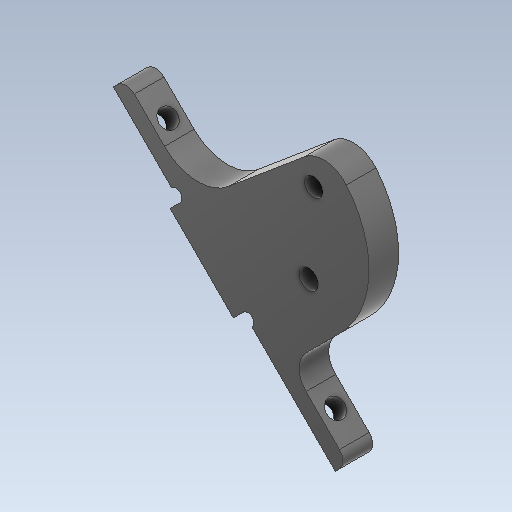
# Autodesk Inventor part: Camera_side_frame
Saved by Autodesk Inventor 2020.4 (Build 244396000, 396)
## iProperties
Created: 2021-09-12
Part Number: Camera_side_frame
Material: アセタール樹脂、黒
Document SubType Name: Modeling
Designer: t-nagamine
Density: 1.425 g/cm^3
Appearance: 滑らか - 黒
Description: POM T5
Mass: 5.16291 g
Surface Area: 23.9114 cm^2
Volume: 3.62309 cm^3
Author: Takuya Nagamine
Autodesk Inventor part; units mm, degrees
ref_plane "YZ Plane" through (0, 0, 0) normal (1, 0, 0) x (0, 1, 0)
ref_plane "XZ Plane" through (0, 0, 0) normal (0, 1, 0) x (-1, 0, 0)
ref_plane "XY Plane" through (0, 0, 0) normal (0, 0, 1) x (1, 0, 0)
derived "Head_side_frame.ipt"
sketch "スケッチ1" plane through (0, 0, 0) normal (0, 0, 1) x (1, 0, 0)
  line L0 (0, 0) -> (27, 0) construction
  line L1 (27, 0) -> (27, 5) construction
  line L2 (27, 5) -> (0, 5) construction
  line L3 (0, 5) -> (0, 0) construction
  line L4 (0, 2.5) -> (27, 2.5) construction
  line L5 (13.5, 5) -> (13.5, 0) construction
  circle A0 centre (3.7, 2.5) radius 1.55
  line L6 (7.5, 5) -> (7.5, 0) construction
  line L7 (19.5, 5) -> (19.5, 0) construction
  circle A1 centre (23.3, 2.5) radius 1.55
  line L8 (7.49, 5.01) -> (9.59, 5.01) construction
  line L9 (19.51, 5.01) -> (19.51, 2.49)
  line L10 (19.51, 2.49) -> (7.49, 2.49)
  line L11 (7.49, 2.49) -> (7.49, 5.01)
  line L12 (7.49, 5.01) -> (19.51, 2.49) construction
  line L13 (19.51, 5.01) -> (7.49, 2.49) construction
  arc A2 (9.59, 5.01) -> (7.49, 5.01) centre (8.54, 5.01) ccw
  arc A3 (19.51, 5.01) -> (17.41, 5.01) centre (18.46, 5.01) ccw
  line L14 (9.59, 5.01) -> (17.41, 5.01)
  line L15 (9.59, 2.49) -> (7.49, 2.49)
  line L16 (17.41, 5.01) -> (19.51, 5.01) construction
  line L17 (27, 7) -> (0, 7) construction
  line L18 (0, 0) -> (0, 7)
  line L19 (12.1912, 40) -> (12.1912, 35) construction
  circle A4 centre (14.8912, 37.5) radius 1.55
  line L20 (37.1912, 35) -> (37.1912, 40) construction
  line L21 (30.6912, 40) -> (30.6912, 35) construction
  circle A5 centre (34.4912, 37.5) radius 1.55
  line L22 (30.7012, 40.01) -> (30.7012, 34.99)
  line L23 (18.6912, 40) -> (18.6912, 35) construction
  line L24 (12.1912, 35) -> (37.1912, 35) construction
  line L25 (37.1912, 40) -> (12.1912, 40) construction
  line L26 (12.1912, 37.5) -> (37.1912, 37.5) construction
  line L27 (24.6912, 40) -> (24.6912, 35) construction
  line L28 (20.7812, 40.01) -> (28.6012, 40.01)
  line L29 (28.6012, 34.99) -> (20.7812, 34.99)
  line L30 (18.6812, 40.01) -> (30.7012, 34.99) construction
  line L31 (30.7012, 40.01) -> (18.6812, 34.99) construction
  arc A6 (30.7012, 40.01) -> (28.6012, 40.01) centre (29.6512, 40.01) ccw
  line L32 (28.6012, 40.01) -> (30.7012, 40.01) construction
  arc A7 (28.6012, 34.99) -> (30.7012, 34.99) centre (29.6512, 34.99) ccw
  line L33 (30.7012, 34.99) -> (28.6012, 34.99) construction
  line L34 (18.6812, 40.01) -> (20.7812, 40.01) construction
  line L35 (20.7812, 34.99) -> (18.6812, 34.99) construction
  arc A8 (20.7812, 40.01) -> (18.6812, 40.01) centre (19.7312, 40.01) ccw
  arc A9 (18.6812, 34.99) -> (20.7812, 34.99) centre (19.7312, 34.99) ccw
  line L36 (18.6812, 34.99) -> (18.6812, 40.01)
  line L37 (18.6912, 73) -> (18.6912, 68) construction
  line L38 (18.6812, 67.99) -> (18.6812, 73.01)
  line L39 (20.7812, 67.99) -> (18.6812, 67.99) construction
  arc A10 (18.6812, 67.99) -> (20.7812, 67.99) centre (19.7312, 67.99) ccw
  arc A11 (20.7812, 73.01) -> (18.6812, 73.01) centre (19.7312, 73.01) ccw
  line L40 (24.6912, 73) -> (24.6912, 68) construction
  line L41 (12.1912, 70.5) -> (37.1912, 70.5) construction
  line L42 (37.1912, 73) -> (12.1912, 73) construction
  line L43 (12.1912, 68) -> (37.1912, 68) construction
  line L44 (30.7012, 73.01) -> (18.6812, 67.99) construction
  line L45 (18.6812, 73.01) -> (30.7012, 67.99) construction
  line L46 (28.6012, 67.99) -> (20.7812, 67.99)
  line L47 (20.7812, 73.01) -> (28.6012, 73.01)
  line L48 (37.1912, 68) -> (37.1912, 73) construction
  line L49 (18.6812, 73.01) -> (20.7812, 73.01) construction
  line L50 (30.6912, 73) -> (30.6912, 68) construction
  arc A12 (30.7012, 73.01) -> (28.6012, 73.01) centre (29.6512, 73.01) ccw
  line L51 (28.6012, 73.01) -> (30.7012, 73.01) construction
  line L52 (30.7012, 73.01) -> (30.7012, 67.99)
  line L53 (30.7012, 67.99) -> (28.6012, 67.99) construction
  circle A13 centre (34.4912, 70.5) radius 1.55
  arc A14 (28.6012, 67.99) -> (30.7012, 67.99) centre (29.6512, 67.99) ccw
  circle A15 centre (14.8912, 70.5) radius 1.55
  line L54 (12.1912, 73) -> (12.1912, 68) construction
  line L55 (27, 0) -> (27, 6.6473)
  line L56 (37.1912, 35) -> (27.1206, 7.3314)
  line L57 (11.8992, 39.6929) -> (0, 7)
  line L58 (37.1912, 35) -> (37.1912, 73)
  line L59 (6.8054, 101.4338) -> (6.7491, 101.3865)
  arc A16 (4.7394, 86.3065) -> (5.3203, 95.7003) centre (-4.8938, 91.617) ccw
  circle A17 centre (-4.8938, 91.617) radius 14.6063 construction
  line L60 (1.0459, 61.9185) -> (-21.5815, 84.5459) construction
  line L61 (-21.5815, 84.5459) -> (-18.0459, 88.0815) construction
  line L62 (-18.0459, 88.0815) -> (4.5815, 65.4541) construction
  line L63 (4.5815, 65.4541) -> (1.0459, 61.9185) construction
  line L64 (1.0459, 61.9185) -> (-18.0459, 88.0815) construction
  line L65 (-21.5815, 84.5459) -> (4.5815, 65.4541) construction
  line L66 (13.8495, 100.8175) -> (37.1912, 73)
  arc A18 (11.8992, 39.6929) -> (5.2055, 80.7796) centre (-28.1256, 54.2607) ccw
  arc A19 (8.344, 97.7899) -> (6.2953, 101.0057) centre (-4.8938, 91.617) ccw construction
  arc A20 (5.0756, 80.942) -> (7.4988, 83.886) centre (-4.8938, 91.617) ccw construction
  circle A21 centre (8.344, 97.7899) radius 1.55
  circle A22 centre (7.4988, 83.886) radius 1.65
  arc A23 (13.8495, 100.8175) -> (6.8054, 101.4338) centre (10.0193, 97.6035) ccw
  arc A24 (6.7491, 101.3865) -> (5.3203, 95.7003) centre (9.9631, 97.5563) ccw
  arc A25 (4.7394, 86.3065) -> (5.2055, 80.7796) centre (9.1182, 83.8926) ccw
  arc A26 (27.1206, 7.3314) -> (27, 6.6473) centre (29, 6.6473) ccw
  arc A27 (7.49, 3.9749) -> (8.9749, 2.49) centre (8.2325, 3.2325) ccw
  arc A28 (18.0251, 2.49) -> (19.51, 3.9749) centre (18.7675, 3.2325) ccw
  line L67 (0, 0) -> (7.5, -0.5)
  line L68 (7.5, -0.5) -> (19.5, -0.5)
  line L69 (27, 0) -> (19.5, -0.5)
  point P0 (24.6912, 37.5)
  point P1 (24.6912, 70.5)
  point P2 (10.6356, 104.6477)
  point P3 (3.5327, 98.6877)
  point P4 (-8.5, 75)
sketch "スケッチ2" plane through (0, 0, 0) normal (0, 0, 1) x (1, 0, 0)
  line L0 (-18.0459, 88.0815) -> (4.5815, 65.4541) construction
  line L1 (12.0061, 58.0294) -> (12.7132, 58.7365)
  line L2 (4.5815, 65.4541) -> (1.0459, 61.9185) construction
  line L3 (-25.4706, 95.5061) -> (-24.7635, 96.2132)
  line L4 (-21.5815, 84.5459) -> (-18.0459, 88.0815) construction
  line L5 (1.0459, 61.9185) -> (-21.5815, 84.5459) construction
  line L6 (-14.1851, 84.2207) -> (-15.8822, 82.5236)
  line L7 (-3.522, 73.5575) -> (-5.219, 71.8604)
  line L8 (-25.4706, 95.5061) -> (-15.6701, 85.7056)
  line L9 (-2.037, 72.0726) -> (12.0061, 58.0294)
  line L10 (-5.219, 71.8604) -> (-15.8822, 82.5236)
  arc A0 (-14.1851, 84.2207) -> (-15.6701, 85.7056) centre (-14.9276, 84.9631) ccw
  arc A1 (-2.037, 72.0726) -> (-3.522, 73.5575) centre (-2.7795, 72.815) ccw
  arc A2 (12.7132, 58.7365) -> (12.7132, 61.565) centre (11.299, 60.1508) ccw
  line L11 (12.7132, 61.565) -> (4.2279, 70.0503)
  line L12 (-11.6606, 85.939) -> (6.8054, 101.4338)
  arc A3 (13.8495, 100.8175) -> (6.8054, 101.4338) centre (10.0193, 97.6035) ccw
  arc A4 (12.8842, 78.7065) -> (13.8495, 100.8175) centre (1.3019, 90.2887) ccw
  line L13 (12.8842, 78.7065) -> (4.2279, 70.0503)
  arc A5 (-21.9348, 96.2132) -> (-24.7635, 96.2132) centre (-23.3491, 94.7989) ccw
  circle A6 centre (7.4988, 83.886) radius 1.65 projected
  circle A7 centre (8.344, 97.7899) radius 1.55 projected
  line L14 (-21.9348, 96.2132) -> (-11.6606, 85.939)
  point P0 (0, 0)
  dimension "d3" = 1
  dimension "d4" = 0
  dimension "d5" = 10.5
  dimension "d6" = 1
  dimension "d7" = 0
  dimension "d8" = 53
  dimension "d9" = 2.4
  dimension "d10" = 15.96
  dimension "d11" = 2.4
  dimension "d12" = 21.96
  dimension "d14" = 2.1
  dimension "d15" = 2.1
  dimension "d17" = 1
  dimension "d18" = 2
  dimension "d23" = 3
  dimension "d29" = 5
  dimension "d42" = 2.0002
  dimension "d43" = 12
  constraints: 22 end point, 12 point on circle, 7 tangent, 6 centre point, 6 perpendicular, 3 parallel, 2 line through centre
  measures "d3" distance of L1.start L1.end
  measures "d4" distance from line of L0 L1.start
  measures "d5" distance between parallel lines of L2 L1
  measures "d6" distance of L3.end L3.start
  measures "d7" distance from line of L3.start L0
  measures "d8" distance between parallel lines of L3 L1
  measures "d9" distance of L6.start L6.end
  measures "d10" distance between parallel lines of L6 L3
  measures "d11" distance of L7.start L7.end
  measures "d12" distance between parallel lines of L1 L7
  measures "d14" distance of L8.end L6.start
  measures "d15" distance of L9.start L7.start
  measures "d17" distance from line of L9 A2.centre
  measures "d18" radius of A2
  measures "d23" distance between parallel lines of L9 L11
  measures "d29" radius of A3
  measures "d42" radius of A5
  measures "d43" distance of L11.start L11.end
extrude "押し出し1" add sketch "スケッチ2" against normal blind 5
sketch "スケッチ4" plane through (-11.6606, 85.939, -5) normal (0.7071068, 0.7071068, 0) x (-0.7071068, 0.7071068, 0)
  line L0 (16.5301, 5) -> (16.5301, 0) projected
  line L1 (-36.4699, 5) -> (-36.4699, 0) projected
  line L2 (2.6701, 0) -> (16.5301, 0) projected
  line L3 (-36.4699, 0) -> (-16.6099, 0) projected
  point P0 (-69.0133, 5)
  point P1 (10.0301, 2.5)
  point P2 (-29.9699, 2.5)
  dimension "d44" = 6.5
  dimension "d45" = 6.5
  dimension "d46" = 2.5
  dimension "d47" = 2.5
  measures "d44" distance from line of point (10.03, 2.5) L0
  measures "d45" distance from line of point (-29.97, 2.5) L1
  measures "d46" distance from line of L2 point (10.03, 2.5)
  measures "d47" distance from line of L3 point (-29.97, 2.5)
hole "穴1" at (-18.7529, 93.0313, -2.5) at (9.5313, 64.7471, -2.5) direction (-0.7071068, -0.7071068, 0) diameter 3.1 end through all
fillet "フィレット1" radius 8 1 edges at (-11.6606, 85.939, -2.5)
fillet "フィレット2" radius 4 1 edges at (4.2279, 70.0503, -2.5)
